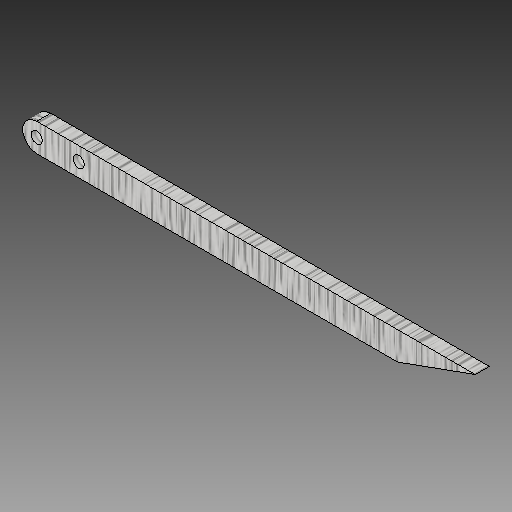
# Autodesk Inventor part: カウンター短
Saved by Autodesk Inventor 2019 (Build 230136000, 136)
## iProperties
Created: 2019-11-14
Part Number: カウンター短
Material: アルミニウム 7075
Document SubType Name: Modeling
Designer: tanjihayato
Density: 2.81 g/cm^3
Appearance: サテン - ブラシ仕上げ 重厚
Mass: 20.2429 g
Surface Area: 46.5964 cm^2
Volume: 7.20388 cm^3
Author: tanjihayato
Autodesk Inventor part; units mm, degrees
ref_plane "YZ Plane" through (0, 0, 0) normal (1, 0, 0) x (0, 1, 0)
ref_plane "XZ Plane" through (0, 0, 0) normal (0, 1, 0) x (-1, 0, 0)
ref_plane "XY Plane" through (0, 0, 0) normal (0, 0, 1) x (1, 0, 0)
sketch "スケッチ1" plane through (0, 0, 0) normal (0, 0, 1) x (1, 0, 0)
  circle A0 centre (0, 0) radius 2
  circle A1 centre (15, 0) radius 2
  arc A2 (0, 5) -> (0, -5) centre (0, 0) ccw
  line L0 (0, 5) -> (156.5134, 5)
  line L1 (156.5134, 5) -> (128.8145, -5)
  line L2 (128.8145, -5) -> (0, -5)
  dimension "d0" = 4
  dimension "d1" = 4
  dimension "d2" = 15
  dimension "d3" = 3
  constraints: 6 end point, 3 centre point, 2 horizontal, 2 point on circle, 2 tangent, 1 coincident, 1 horizontal alignment
  measures "d0" diameter of A0
  measures "d1" diameter of A1
  measures "d2" distance of A1.centre point (0, 0)
  measures "d3" radial gap between concentric circles of A0 A2
extrude "押し出し1" add sketch "スケッチ1" along normal blind 5
